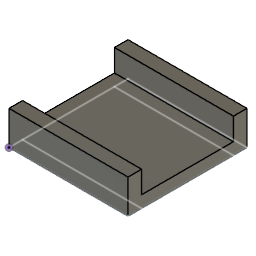
display_spacer (Autodesk Fusion 360 design; units mm, degrees)
Autodesk Fusion 360 part; units mm, degrees
sketch "Sketch1" plane through (0, 0, 0) normal (0, 0, 1) x (1, 0, 0)
  line L0 (0, 0) -> (14, 0)
  line L1 (14, 0) -> (14, 14)
  line L2 (14, 14) -> (0, 14)
  line L3 (0, 14) -> (0, 0)
  line L4 (0, 12.4) -> (14, 12.4)
  line L5 (0, 1.6) -> (14, 1.6)
  dimension "d1" = 14
  dimension "d2" = 14
  dimension "d3" = 1.6
  dimension "d4" = 1.6
  constraint horizontal L0
  constraint vertical L1
  constraint horizontal L2
  constraint vertical L3
  constraint coincident L0.start L3.end
  constraint coincident L3 L4.start
  constraint coincident L1 L4.end
  constraint perpendicular L1 L4
  constraint coincident L3 L5.start
  constraint coincident L1 L5.end
  constraint perpendicular L1 L5
  measures "d1" distance of L0.start L0.end
  measures "d2" distance of L0.start L2.end
  measures "d3" distance of L2 L4
  measures "d4" distance of L0 L5
extrude "Extrude1" add sketch "Sketch1" along normal blind 1.4
extrude "Extrude2" add sketch "Sketch1" along normal blind 4 contours L0 L1 L3 L5 | L1 L2 L3 L4
